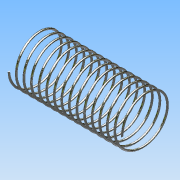
# Autodesk Inventor part: Shock Spring
Saved by Autodesk Inventor 2015 (Build 190159000, 159)
## iProperties
Created: 2014-01-04
Part Number: Shock Spring
Material: Stainless Steel
Document SubType Name: Modeling
Designer: davidgitz
Density: 8.08 g/cm^3
Appearance: Chrome - Polished
Author: davidgitz
Autodesk Inventor part; units mm, degrees
ref_plane "YZ Plane" through (0, 0, 0) normal (1, 0, 0) x (0, 1, 0)
ref_plane "XZ Plane" through (0, 0, 0) normal (0, 1, 0) x (-1, 0, 0)
ref_plane "XY Plane" through (0, 0, 0) normal (0, 0, 1) x (1, 0, 0)
sketch "Sketch1" plane through (0, 0, 0) normal (1, 0, 0) x (0, 1, 0)
  circle A0 centre (0, 0) radius 8.509
  dimension "d0" = 17.018
  constraints: 1 centre point, 1 coincident
  measures "d0" diameter of A0
extrude "Extrusion1" add sketch "Sketch1" along normal blind 38.1
sketch "Sketch3" plane through (0, 0, 0) normal (0, 1, 0) x (-1, 0, 0)
  line L0 (0, 8.509) -> (-38.1, 8.509) projected
  line L1 (0, -8.509) -> (0, 8.509) projected
  circle A0 centre (0, 8.1915) radius 0.3175
  point P0 (0, 0)
  dimension "d12" = 0.635
  constraints: 1 centre point, 1 point on line, 1 tangent
  measures "d12" diameter of A0
coil "Coil2" sketch "Sketch3" operation intersect axis through (-10, 0, 0) along (1, 0, 0) pitch 2.54 turns 15 hand right
equation "\"d13\" = 0.0666667 * HEIGHT"
equation "\"d14\" = HEIGHT"
equation "\"HEIGHT\" = 38.1"
body "Solid1"
